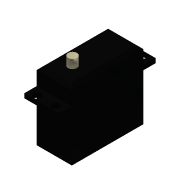
# Autodesk Inventor part: Servo_Drehwerk
Saved by Autodesk Inventor 2015 (Build 190159000, 159)
## iProperties
Created: 2014-12-18
Part Number: Servo_Drehwerk
Material: Aluminium 6061
Document SubType Name: Modeling
Designer: Luki
Density: 2.7 g/cm^3
Appearance: Eloxiert - schwarz
Mass: 86.3708 g
Surface Area: 69.0823 cm^2
Volume: 31.9892 cm^3
Author: Luki
Autodesk Inventor part; units mm, degrees
ref_plane "YZ Plane" through (0, 0, 0) normal (1, 0, 0) x (0, 1, 0)
ref_plane "XZ Plane" through (0, 0, 0) normal (0, 1, 0) x (-1, 0, 0)
ref_plane "XY Plane" through (0, 0, 0) normal (0, 0, 1) x (1, 0, 0)
sketch "Skizze1" plane through (0, 0, 0) normal (0, 0, 1) x (1, 0, 0)
  line L0 (-10, -20.3) -> (10, -20.3)
  line L1 (10, -20.3) -> (10, 20.3)
  line L2 (10, 20.3) -> (-10, 20.3)
  line L3 (-10, 20.3) -> (-10, -20.3)
  line L4 (-10, -20.3) -> (10, 20.3) construction
  line L5 (10, -20.3) -> (-10, 20.3) construction
  point P0 (0, 0)
  dimension "d0" = 20
  dimension "d1" = 40.6
  constraints: 12 end point, 2 midpoint, 2 parallel, 1 horizontal, 1 perpendicular
  measures "d0" distance between parallel lines of L3 L1
  measures "d1" distance between parallel lines of L0 L2
extrude "Extrusion1" add sketch "Skizze1" along normal blind 26.5
sketch "Skizze2" plane through (0, 0, 26.5) normal (0, 0, 1) x (1, 0, 0)
  point P0 (0, 0)
sketch "Skizze3" plane through (0, 0, 26.5) normal (0, 0, 1) x (1, 0, 0)
  line L0 (-10, 20.3) -> (-10, -20.3) projected
  line L1 (10, -20.3) -> (10, 20.3) projected
  line L2 (10, 20.3) -> (-10, 20.3) projected
  line L3 (-10, -20.3) -> (10, -20.3) projected
  line L4 (-10, -27.25) -> (10, -27.25)
  line L5 (10, -27.25) -> (10, 27.25)
  line L6 (10, 27.25) -> (-10, 27.25)
  line L7 (-10, 27.25) -> (-10, -27.25)
  line L8 (-10, -27.25) -> (10, 27.25) construction
  line L9 (10, -27.25) -> (-10, 27.25) construction
  point P0 (0, 0)
  dimension "d4" = 54.5
  dimension "d5" = 0
  constraints: 12 end point, 2 midpoint, 2 parallel, 1 horizontal, 1 perpendicular
  measures "d4" distance between parallel lines of L4 L6
  measures "d5" distance between parallel lines of L0 L7
extrude "Extrusion2" add sketch "Skizze3" along normal blind 2.5
sketch "Skizze4" plane through (0, 0, 29) normal (0, 0, 1) x (1, 0, 0)
  line L0 (10, -20.3) -> (10, 20.3) projected
  line L1 (-10, -20.3) -> (10, -20.3)
  line L2 (10, -20.3) -> (10, 20.3)
  line L3 (10, 20.3) -> (-10, 20.3)
  line L4 (-10, 20.3) -> (-10, -20.3)
  line L5 (-10, -20.3) -> (10, 20.3) construction
  line L6 (10, -20.3) -> (-10, 20.3) construction
  point P0 (0, 0)
  dimension "d8" = 40.6
  constraints: 12 end point, 2 midpoint, 2 parallel, 1 horizontal, 1 perpendicular, 1 point on line
  measures "d8" distance between parallel lines of L1 L3
extrude "Extrusion3" add sketch "Skizze4" along normal blind 9.9
sketch "Skizze6" plane through (0, 0, 29) normal (0, 0, 1) x (1, 0, 0)
  line L0 (10, -27.25) -> (-10, -27.25) projected
  line L1 (-10, -27.25) -> (-10, -20.3) projected
  line L2 (10, -20.3) -> (-10, -20.3) projected
  line L3 (10, 20.3) -> (10, -20.3) projected
  line L4 (-10, 20.3) -> (10, 20.3) projected
  line L5 (-10, 20.3) -> (-10, 27.25) projected
  line L6 (-10, 27.25) -> (10, 27.25) projected
  line L7 (10, 27.25) -> (10, 20.3) projected
  line L8 (10, -20.3) -> (10, -27.25) projected
  line L9 (-10, -20.3) -> (-10, 20.3) projected
  circle A0 centre (5, 24.75) radius 2.25
  line L10 (-14, 0) -> (14, 0) projected
  line L11 (0, 38.15) -> (0, -38.15) projected
  point P0 (0, 0)
  dimension "d12" = 24.75
  dimension "d13" = 5
  dimension "d14" = 4.5
  constraints: 1 centre point
  measures "d12" distance from line of A0.centre L10
  measures "d13" distance from line of A0.centre L11
  measures "d14" diameter of A0
extrude "Extrusion4" cut sketch "Skizze6" against normal blind 9.9 contours A0
mirror "Spiegeln1" about plane through (0, 0, 0) normal (0, 1, 0) of "Extrusion4"
mirror "Spiegeln2" about plane through (0, 0, 0) normal (1, 0, 0) of "Extrusion4", "Spiegeln1"
sketch "Skizze7" plane through (0, 0, 38.9) normal (0, 0, 1) x (1, 0, 0)
  line L0 (0, 38.15) -> (0, -38.15) projected
  line L1 (-14, 0) -> (14, 0) projected
  circle A0 centre (-5, -24.75) radius 2.25 projected
  circle A1 centre (5, -24.75) radius 2.25 projected
  circle A2 centre (0, -9.9) radius 2.5
  point P0 (0, 0)
  dimension "d18" = 14.85
  dimension "d19" = 5
  constraints: 1 centre point, 1 point on line
  measures "d18" vertical distance of A0.centre A2.centre
  measures "d19" diameter of A2
extrude "Extrusion5" add sketch "Skizze7" along normal blind 5 contours A2 L0 | L0 A2
chamfer "Fase1" distance 2 angle 45 4 edges at (0, -20.3, 38.9) (0, 20.3, 38.9) (10, 0, 38.9) (-10, 0, 38.9)
